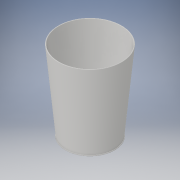
# Autodesk Inventor part: trash bin 13 inches not demanding
Saved by Autodesk Inventor 2017 (Build 210142000, 142)
## iProperties
Created: 2018-03-23
Part Number: trash bin 13 inches not demanding
Material: Generic
Document SubType Name: Modeling
Designer: braxtonwright
Density: 1 g/cm^3
Appearance: Default
Author: braxtonwright
Autodesk Inventor part; units mm, degrees
ref_plane "YZ Plane" through (0, 0, 0) normal (1, 0, 0) x (0, 1, 0)
ref_plane "XZ Plane" through (0, 0, 0) normal (0, 1, 0) x (-1, 0, 0)
ref_plane "XY Plane" through (0, 0, 0) normal (0, 0, 1) x (1, 0, 0)
sketch "Sketch1" plane through (0, 0, 0) normal (0, 0, 1) x (1, 0, 0)
  line L0 (0, 0) -> (8.4667, 0) construction
  arc A0 (8.4667, -0.1519) -> (8.4667, 0.1519) centre (8.4667, 0) ccw
  line L1 (8.4667, -0.1519) -> (0, -0.1519)
  line L2 (0, -0.1519) -> (0, 0)
  line L3 (8.4667, 0.1519) -> (0, 0.1519)
  line L4 (0, 0.1519) -> (0, 0)
  dimension "d0" = 8.4667
  dimension "d1" = 0.3037
  dimension "d2" = 8.4667
  dimension "d3" = 8.4667
  constraints: 10 end point, 3 perpendicular, 2 point on circle, 1 centre point, 1 coincident, 1 horizontal, 1 parallel, 1 point on line
  measures "d0" distance of L0.start L0.end
  measures "d1" diameter of A0
  measures "d2" distance of L3.start L3.end
  measures "d3" distance of L1.start L1.end
revolve "bace" add sketch "Sketch1" angle 360 about axis through (0, 0.1519, 0) along (0, -1, 0)
sketch "Sketch2" plane through (0, 0, 0) normal (1, 0, 0) x (0, 1, 0)
  line L0 (0.1519, 8.4667) -> (0.1519, -8.4667) projected
  line L1 (0.1519, 0) -> (27.6685, 0)
  line L2 (27.6685, 0) -> (27.6685, -11.0747)
  line L3 (27.6685, -11.0747) -> (0.1519, -8.4667)
  line L4 (27.6685, -11.0747) -> (27.6685, -10.7709)
  line L5 (27.6685, -10.7709) -> (0.1519, -8.1629)
  line L6 (0.1519, -8.4667) -> (0.1519, -8.1629)
  point P0 (0, 0)
  dimension "d5" = 27.5167
  dimension "d6" = 0.3037
  dimension "d7" = 0.3037
  constraints: 12 end point, 2 point on line, 1 collinear, 1 horizontal, 1 midpoint, 1 parallel, 1 perpendicular
  measures "d5" distance of L1.start L1.end
  measures "d6" distance of L2.end L4.end
  measures "d7" distance of L0.end L5.end
revolve "walls" add sketch "Sketch2" angle 360 about axis through (0, 0.1519, 0) along (0, 1, 0) contours L5 L2 L3 L0
sketch "Sketch3" plane through (0, 0, 0) normal (0, 0, 1) x (1, 0, 0)
  line L0 (8.1629, 0.1519) -> (10.7709, 27.6685) projected
  line L1 (10.7709, 27.6685) -> (11.0747, 27.6685) construction
  line L2 (11.0747, 27.6685) -> (8.4667, 0.1519) projected
  line L3 (-11.0747, 27.6685) -> (11.0747, 27.6685) projected
  arc A0 (11.0747, 27.6685) -> (10.7709, 27.6685) centre (10.9228, 27.6685) ccw
  line L4 (0, -5.7418) -> (0, 33.3874) projected
  point P0 (0, 0)
  dimension "d10" = 0.1519
  constraints: 2 end point, 2 point on circle, 2 point on line, 1 centre point, 1 horizontal
  measures "d10" radius of A0
revolve "Revolution3" add sketch "Sketch3" angle 360 about axis through (0, -10, 0) along (0, 1, 0)
equation "\"d2\" = d0"
equation "\"d3\" = d0"
equation "\"d6\" = d1"
equation "\"d10\" = 0.5 * d1"
body "Solid1"
